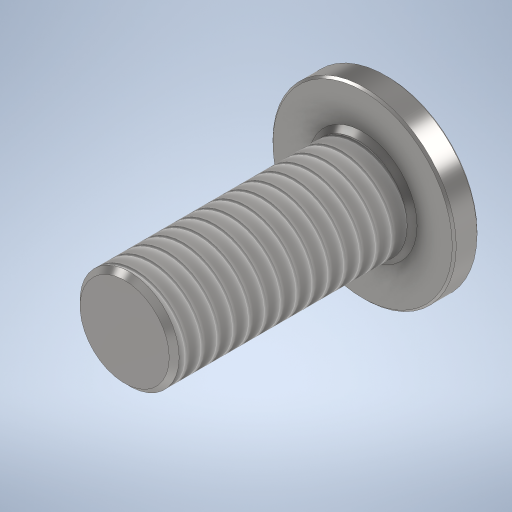
# Autodesk Inventor part: Low Profile M5x12
Saved by Autodesk Inventor 2024 (Build 280153000, 153)
## iProperties
Created: 2024-09-05
Part Number: Low Profile M5x12
Material: Stainless Steel
Document SubType Name: Modeling
Designer: Ishaan
Density: 8 g/cm^3
Appearance: Semi-Polished
Author: Ishaan
Autodesk Inventor part; units mm, degrees
ref_plane "YZ Plane" through (0, 0, 0) normal (1, 0, 0) x (0, 1, 0)
ref_plane "XZ Plane" through (0, 0, 0) normal (0, 1, 0) x (-1, 0, 0)
ref_plane "XY Plane" through (0, 0, 0) normal (0, 0, 1) x (1, 0, 0)
sketch "Sketch1" plane through (0, 0, 0) normal (0, 0, 1) x (1, 0, 0)
  circle A0 centre (0, 0) radius 4.625
  circle A1 centre (0, 0) radius 2.5
  dimension "d0" = 9.25
  dimension "d1" = 5
  constraints: 2 centre point, 2 coincident
  measures "d0" diameter of A0
  measures "d1" diameter of A1
extrude "Extrusion1" add sketch "Sketch1" along normal blind 12 contours A1
extrude "Extrusion2" add sketch "Sketch1" against normal blind 1.25 contours A0 | A1
thread "Thread1" size "M5x0.8" class "6g" standard "ANSI Metric M Profile" full length
chamfer "Chamfer1" distance 0.1 angle 45 2 edges at (-4.625, 0, 0) (-4.625, 0, -1.25)
sketch "Sketch2" plane through (0, 0, -1.25) normal (0, 0, -1) x (-1, 0, 0)
  circle A0 centre (0, 0) radius 1.97 construction
  line L0 (1.64, 0) -> (0.82, -1.4203) construction
  line L1 (0.82, -1.4203) -> (-0.82, -1.4203) construction
  line L2 (-0.82, -1.4203) -> (-1.64, 0) construction
  line L3 (-1.64, 0) -> (-0.82, 1.4203) construction
  line L4 (-0.82, 1.4203) -> (0.82, 1.4203) construction
  line L5 (0.82, 1.4203) -> (1.64, 0) construction
  circle A1 centre (1.64, 0) radius 0.33
  circle A2 centre (0.82, -1.4203) radius 0.33
  circle A3 centre (-0.82, -1.4203) radius 0.33
  circle A4 centre (-1.64, 0) radius 0.33
  circle A5 centre (-0.82, 1.4203) radius 0.33
  circle A6 centre (0.82, 1.4203) radius 0.33
  circle A7 centre (1.9406, 1.1204) radius 0.83
  circle A8 centre (1.9406, -1.1204) radius 0.83
  circle A9 centre (0, -2.2408) radius 0.83
  circle A10 centre (-1.9406, -1.1204) radius 0.83
  circle A11 centre (-1.9406, 1.1204) radius 0.83
  circle A12 centre (0, 2.2408) radius 0.83
  circle A13 centre (0, 0) radius 1.25
  point P0 (-0.5867, 1.6537)
  point P1 (-1.1388, 1.335)
  point P2 (-1.7255, 0.3187)
  point P3 (-1.7255, -0.3187)
  point P4 (-1.1388, -1.335)
  point P5 (-0.5867, -1.6537)
  point P6 (0.5867, -1.6537)
  point P7 (1.1388, -1.335)
  point P8 (1.7255, -0.3187)
  point P9 (1.7255, 0.3187)
  point P10 (1.1388, 1.335)
  point P11 (0.5867, 1.6537)
  dimension "d30" = 3.94
  dimension "d31" = 0.66
  dimension "d32" = 1.66
  dimension "d33" = 2.5
  constraints: 14 centre point, 13 tangent, 12 end point, 10 equal radius, 9 coincident, 1 horizontal, 13 other
  measures "d30" diameter of A0
  measures "d31" diameter of A1
  measures "d32" diameter of A7
  measures "d33" diameter of A13
hole "Hole1" at (0, 0, -1.25) direction (0, 0, 1) diameter 2.5 depth 2.5 tip angle 150
chamfer "Chamfer2" distance 0.5 distance2 0.8 1 edges at (0, -1.25, -1.25) measured on face at (0, -1.25, -0.75)
extrude "Extrusion4" cut sketch "Sketch2" against normal up to surface contours A1 | A1 A8 A2 A9 A3 A10 A4 A11 A5 A12 A6 A7 | A6 | A2 | A5 | A3 | A4 | A13 round surface about axis through (0, 0, 1.4175) along (0, 0, -1) radius 0.625 half angle 75 far side no
chamfer "Chamfer3" distance 0.25 angle 45 2 edges at (-2.5, 0, 0) (-2.5, 0, 12)
equation "\"d23\" = d33"
body "Solid1"
